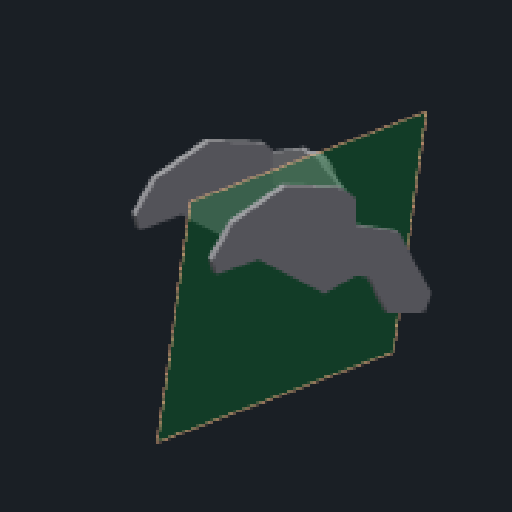
# Autodesk Inventor part: ShoulderCollision
Saved by Autodesk Inventor 2025.2 (Build 292293000, 293)
## iProperties
Created: 2023-03-28
Part Number: ShoulderCollision
Material: Generic
Document SubType Name: Modeling
Designer: LattePanda
Density: 1 g/cm^3
Appearance: Default
Author: LattePanda
Autodesk Inventor part; units mm, degrees
sketch "Sketch1" plane through (0, 0, 0) normal (0, 0, 1) x (1, 0, 0)
  circle A0 centre (0, 0) radius 14
  arc A1 (-9.6844, 3.0721) -> (-9.6844, -3.0721) centre (0, 0) ccw construction
  circle A2 centre (0, 0) radius 14
  constraints: 2 centre point, 1 coincident, 1 concentric, 2 other
ref_plane "Work Plane1" through (-24.1297, -20.1241, 6.985) normal (0, 0, -1) x (0, 1, 0)
extrude "Extrusion1" add sketch "Sketch1" along normal up to surface (6.985 mm away)
sketch "Sketch2" plane through (0, 0, 6.985) normal (0, 0, 1) x (1, 0, 0)
  line L0 (24.1297, -19.05) -> (-24.1297, -19.05) construction
  line L1 (30.4797, -4.9571) -> (30.4797, -51.5313) construction
  line L2 (-30.4797, -51.5313) -> (-30.4797, -4.9571) construction
  line L3 (-6.5797, 18.2867) -> (-30.4797, 3.81)
  line L4 (6.5797, 18.2867) -> (30.4797, 3.81)
  line L5 (30.4797, 3.81) -> (30.4797, -19.05)
  line L6 (30.4797, -19.05) -> (-30.4797, -19.05)
  line L7 (-30.4797, -19.05) -> (-30.4797, 3.81)
  line L8 (0, 141.501) -> (0, -68.047)
  arc A0 (6.5797, 18.2867) -> (-6.5797, 18.2867) centre (0, 7.4241) ccw construction
  line L9 (6.5797, 18.2867) -> (24.1297, 7.6563) construction
  line L10 (-24.1297, 7.6563) -> (-6.5797, 18.2867) construction
  line L11 (6.5797, 18.2867) -> (-6.5797, 18.2867)
  point P0 (0, 0)
  point P1 (0, -5.2759)
  point P2 (-30.4797, 16.6942)
  point P3 (-5.3196, -19.05)
  constraints: 14 end point, 5 collinear, 2 perpendicular, 2 vertical, 1 horizontal, 1 point on line, 2 other
ref_plane "Work Plane2" through (-24.1297, -20.1241, 10.16) normal (0, 0, 1) x (1, 0, 0)
extrude "Extrusion2" add sketch "Sketch2" along normal up to surface (3.175 mm away)
ref_plane "Work Plane3" through (30.4797, -27.7824, 45.9277) normal (-1, 0, 0) x (0, -0.986, 0.1668)
sketch "Sketch3" plane through (30.4797, -27.7824, 45.9277) normal (-1, 0, 0) x (0, -0.986, 0.1668)
  line L0 (-47.9068, 72.7646) -> (-31.8636, 83.3523) construction
  line L1 (-25.5087, 83.7046) -> (-20.9193, 81.3584) construction
  line L2 (-17.4786, 75.8356) -> (-17.0001, 46.1314) construction
  line L3 (-61.535, 29.6482) -> (-50.5122, 69.1886) construction
  line L4 (-45.3902, -22.2294) -> (-61.4405, 25.9552) construction
  line L5 (-15.9257, 42.7078) -> (21.8176, -13.4116) construction
  line L6 (24.78, -27.1582) -> (21.9473, -43.9057) construction
  line L7 (-18.293, -38.7417) -> (-32.0753, -36.4163) construction
  line L8 (-35.8826, -34.2371) -> (-44.4025, -24.0864) construction
  line L9 (1.5345, -78.0839) -> (-13.5009, -42.5299) construction
  line L10 (52.2811, -114.2632) -> (3.7676, -80.8246) construction
  line L11 (22.2253, -47.0922) -> (25.3496, -55.8788) construction
  line L12 (27.7289, -58.9798) -> (55.688, -78.2509) construction
  line L13 (58.1761, -81.7138) -> (65.2363, -106.3801) construction
  line L14 (60.9015, -114.1914) -> (57.6044, -115.1351) construction
  line L15 (-49.878, 71.4637) -> (-28.7889, 85.3815)
  line L16 (-28.7889, 85.3815) -> (-17.5398, 79.6307)
  line L17 (-17.5398, 79.6307) -> (-16.9699, 44.2605)
  line L18 (-16.9699, 44.2605) -> (26.0426, -19.6937)
  line L19 (26.0426, -19.6937) -> (21.6717, -45.5351)
  line L20 (21.6717, -45.5351) -> (26.0378, -57.8141)
  line L21 (26.0378, -57.8141) -> (57.5529, -79.5363)
  line L22 (57.5529, -79.5363) -> (66.9746, -112.4531)
  line L23 (66.9746, -112.4531) -> (54.7369, -115.9559)
  line L24 (54.7369, -115.9559) -> (2.2516, -79.7797)
  line L25 (2.2516, -79.7797) -> (-14.8578, -39.3213)
  line L26 (-14.8578, -39.3213) -> (-34.38, -36.0274)
  line L27 (-34.38, -36.0274) -> (-45.0145, -23.3573)
  line L28 (-45.0145, -23.3573) -> (-62.0524, 27.7923)
  line L29 (-62.0524, 27.7923) -> (-49.878, 71.4637)
  point P0 (-35.053, -40.651)
  point P1 (21.6748, -26.5696)
  point P2 (-49.9314, -21.2415)
  point P3 (-37.7332, 79.4786)
  constraints: 30 end point, 15 collinear, 1 parallel
ref_plane "Work Plane4" through (-33.6547, -38.1116, -58.8269) normal (-1, 0, 0) x (0, 0.0012, 1)
extrude "Extrusion4" add sketch "Sketch3" against normal blind 4
mirror "Mirror1" about plane through (0, 0, 0) normal (1, 0, 0) of "Extrusion4"
body "Solid1"
